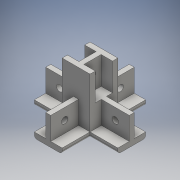
# Autodesk Inventor part: fourwaylockver1
Saved by Autodesk Inventor 2016 (Build 200138000, 138)
## iProperties
Created: 2015-11-21
Part Number: fourwaylockver1
Material: Generic
Document SubType Name: Modeling
Designer: hesaon
Density: 1 g/cm^3
Appearance: Default
Author: hesaon
Autodesk Inventor part; units mm, degrees
ref_plane "YZ Plane" through (0, 0, 0) normal (1, 0, 0) x (0, 1, 0)
ref_plane "XZ Plane" through (0, 0, 0) normal (0, 1, 0) x (-1, 0, 0)
ref_plane "XY Plane" through (0, 0, 0) normal (0, 0, 1) x (1, 0, 0)
sketch "Sketch1" plane through (0, 0, 0) normal (0, 0, 1) x (1, 0, 0)
  line L0 (0, 0) -> (20, 0)
  line L1 (20, 0) -> (20, 20)
  line L2 (20, 20) -> (0, 20)
  line L3 (0, 20) -> (0, 0)
  line L4 (0, 0) -> (20, 0)
  line L5 (20, 0) -> (20, -20)
  line L6 (20, -20) -> (0, -20)
  line L7 (0, -20) -> (0, 0)
  line L8 (20, 0) -> (40, 0)
  line L9 (40, 0) -> (40, -20)
  line L10 (40, -20) -> (20, -20)
  line L11 (20, -20) -> (20, 0)
  line L12 (0, -20) -> (-20, -20)
  line L13 (-20, -20) -> (-20, 0)
  line L14 (-20, 0) -> (0, 0)
  line L15 (0, 0) -> (0, -20)
  line L16 (0, -20) -> (20, -20)
  line L17 (20, -20) -> (20, -40)
  line L18 (20, -40) -> (0, -40)
  line L19 (0, -40) -> (0, -20)
  dimension "d0" = 20
  dimension "d1" = 20
  dimension "d2" = 20
  dimension "d3" = 20
  dimension "d4" = 20
  dimension "d5" = 20
  dimension "d6" = 20
  dimension "d7" = 20
  dimension "d8" = 20
  dimension "d9" = 20
  constraints: 40 end point, 10 parallel, 5 horizontal, 5 perpendicular
  measures "d0" distance of L2.end L1.end
  measures "d1" distance of L1.end L0.end
  measures "d2" distance of L5.end L6.end
  measures "d3" distance of L4.end L5.end
  measures "d4" distance of L9.end L10.end
  measures "d5" distance of L8.end L9.end
  measures "d6" distance of L13.end L14.end
  measures "d7" distance of L12.end L13.end
  measures "d8" distance of L17.end L18.end
  measures "d9" distance of L16.end L17.end
extrude "Extrusion1" add sketch "Sketch1" along normal blind 3.8
sketch "Sketch2" plane through (0, 0, 3.8) normal (0, 0, 1) x (1, 0, 0)
  line L0 (-20, 0) -> (-20, -20) projected
  line L1 (-20, -8.2) -> (0, -8.2)
  line L2 (0, -8.2) -> (0, -11.8)
  line L3 (0, -11.8) -> (-20, -11.8)
  line L4 (-20, -11.8) -> (-20, -8.2)
  line L5 (-20, -20) -> (0, -20) projected
  line L6 (0, 0) -> (20, 0)
  line L7 (20, 0) -> (20, -20)
  line L8 (20, -20) -> (0, -20)
  line L9 (0, -20) -> (0, 0)
  line L10 (40, -20) -> (40, 0) projected
  line L11 (20, -8.2) -> (40, -8.2)
  line L12 (40, -8.2) -> (40, -11.8)
  line L13 (40, -11.8) -> (20, -11.8)
  line L14 (20, -11.8) -> (20, -8.2)
  line L15 (20, 20) -> (0, 20) projected
  line L16 (8.2, 0) -> (11.8, 0)
  line L17 (11.8, 0) -> (11.8, 20)
  line L18 (11.8, 20) -> (8.2, 20)
  line L19 (8.2, 20) -> (8.2, 0)
  line L20 (0, -40) -> (20, -40) projected
  line L21 (8.2, -20) -> (11.8, -20)
  line L22 (11.8, -20) -> (11.8, -40)
  line L23 (11.8, -40) -> (8.2, -40)
  line L24 (8.2, -40) -> (8.2, -20)
  dimension "d12" = 8.2
  dimension "d13" = 8.2
  dimension "d14" = 20
  dimension "d15" = 8.2
  dimension "d16" = 8.2
  dimension "d17" = 8.2
  dimension "d18" = 8.2
  dimension "d19" = 8.2
  dimension "d20" = 8.2
  constraints: 40 end point, 10 parallel, 7 point on line, 5 horizontal, 5 perpendicular
  measures "d12" distance of L0.start L1.start
  measures "d13" distance between parallel lines of L3 L5
  measures "d14" distance of L1.end L1.start
  measures "d15" distance of L11.end L10.end
  measures "d16" distance of L12.end L10.start
  measures "d17" distance of L18.end L15.end
  measures "d18" distance of L15.start L17.end
  measures "d19" distance of L20.end L22.end
  measures "d20" distance of L20.start L23.end
extrude "Extrusion2" add sketch "Sketch2" along normal blind 16.2 contours L1 L2 L3 L0 | L9 L6 L7 L8 L2 | L19 L15 L17 L6 | L8 L22 L20 L24 | L11 L10 L13 L7
sketch "Sketch3" plane through (0, 0, 20) normal (0, 0, 1) x (1, 0, 0)
  line L0 (0, 0) -> (0, -8.2) projected
  line L1 (0, 0) -> (0, -3.8)
  line L2 (0, -3.8) -> (8.2, -3.8)
  line L3 (8.2, -3.8) -> (8.2, -16.2)
  line L4 (8.2, -16.2) -> (0, -16.2)
  line L5 (0, -11.8) -> (0, -20) projected
  line L6 (0, -16.2) -> (0, -20)
  line L7 (20, -40) -> (20, -20) projected
  line L8 (0, -20) -> (20, -20)
  line L9 (20, -20) -> (20, -16.2)
  line L10 (20, -20) -> (20, -11.8) projected
  line L11 (20, -16.2) -> (11.8, -16.2)
  line L12 (11.8, -16.2) -> (11.8, -3.8)
  line L13 (11.8, -3.8) -> (20, -3.8)
  line L14 (20, -8.2) -> (20, 0) projected
  line L15 (8.2, 0) -> (0, 0) projected
  line L16 (20, 0) -> (0, 0)
  line L17 (40, 0) -> (20, 0) projected
  line L18 (20, 0) -> (20, -3.8)
  dimension "d23" = 3.8
  dimension "d24" = 8.2
  dimension "d25" = 12.4
  dimension "d26" = 8.2
  constraints: 24 end point, 8 point on line, 5 perpendicular, 3 collinear
  measures "d23" distance of L0.start L1.end
  measures "d24" distance of L1.end L2.end
  measures "d25" distance of L2.end L3.end
  measures "d26" distance of L9.end L11.end
extrude "Extrusion3" add sketch "Sketch3" along normal blind 19.8
sketch "Sketch4" plane through (11.8, 0, 3.8) normal (1, 0, 0) x (0, 0, -1)
  circle A0 centre (-8.2, 10) radius 2.25
  line L0 (-16.2, 0) -> (-16.2, 20) projected
  line L1 (0, 20) -> (-16.2, 20) projected
  point P0 (3.8, 0)
  dimension "d29" = 4.5
  dimension "d30" = 8
  dimension "d31" = 10
  constraints: 1 centre point
  measures "d29" diameter of A0
  measures "d30" distance from line of L0 A0.centre
  measures "d31" distance from line of L1 A0.centre
extrude "Extrusion4" cut sketch "Sketch4" against normal through all
sketch "Sketch5" plane through (11.8, -40, 3.8) normal (1, 0, 0) x (0, 0, -1)
  circle A0 centre (-8.2, 10) radius 2.25
  line L0 (-16.2, 0) -> (-16.2, 20) projected
  line L1 (0, 0) -> (-16.2, 0) projected
  point P0 (3.8, 40)
  dimension "d34" = 4.5
  dimension "d35" = 8
  dimension "d36" = 10
  constraints: 1 centre point
  measures "d34" diameter of A0
  measures "d35" distance from line of L0 A0.centre
  measures "d36" distance from line of L1 A0.centre
extrude "Extrusion5" cut sketch "Sketch5" against normal through all
sketch "Sketch6" plane through (11.8, -16.2, 20) normal (1, 0, 0) x (0, 0, -1)
  circle A0 centre (-10, 6.2) radius 2.25
  line L0 (0, 4.4) -> (0, 8) projected
  line L1 (16.2, 16.2) -> (-19.8, 16.2) projected
  point P0 (20, 16.2)
  dimension "d39" = 4.5
  dimension "d40" = 10
  dimension "d41" = 10
  constraints: 1 centre point
  measures "d39" diameter of A0
  measures "d40" distance from line of L0 A0.centre
  measures "d41" distance from line of L1 A0.centre
extrude "Extrusion6" cut sketch "Sketch6" against normal through all
sketch "Sketch7" plane through (20, -11.8, 3.8) normal (0, -1, 0) x (1, 0, 0)
  circle A0 centre (10, 8.2) radius 2.25
  line L0 (0, 16.2) -> (20, 16.2) projected
  line L1 (20, 0) -> (20, 16.2) projected
  point P0 (-20, -3.8)
  dimension "d44" = 4.5
  dimension "d45" = 8
  dimension "d46" = 10
  constraints: 1 centre point
  measures "d44" diameter of A0
  measures "d45" distance from line of L0 A0.centre
  measures "d46" distance from line of L1 A0.centre
extrude "Extrusion7" cut sketch "Sketch7" against normal through all
sketch "Sketch8" plane through (-20, -11.8, 3.8) normal (0, -1, 0) x (1, 0, 0)
  circle A0 centre (10, 8.2) radius 2.25
  line L0 (0, 16.2) -> (20, 16.2) projected
  line L1 (0, 0) -> (0, 16.2) projected
  point P0 (20, -3.8)
  dimension "d49" = 4.5
  dimension "d50" = 8
  dimension "d51" = 10
  constraints: 1 centre point
  measures "d49" diameter of A0
  measures "d50" distance from line of L0 A0.centre
  measures "d51" distance from line of L1 A0.centre
extrude "Extrusion8" cut sketch "Sketch8" against normal through all
fillet "Fillet1" radius 2 8 edges at (-10, 0, 0) (0, 10, 0) (-10, -20, 0) (0, -30, 0) (20, -30, 0) (30, -20, 0) (30, 0, 0) (20, 10, 0)
equation "\"d13\" = d12"
equation "\"d15\" = d12"
equation "\"d16\" = d12"
equation "\"d17\" = d12"
equation "\"d18\" = d12"
equation "\"d19\" = d12"
equation "\"d20\" = d12"
equation "\"d26\" = d24"
body "Solid1"
